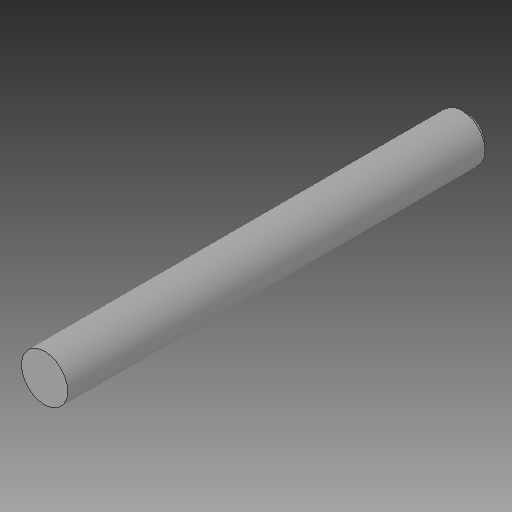
# Autodesk Inventor part: trappestift
Saved by Autodesk Inventor 2018 (Build 220112000, 112)
## iProperties
Created: 2019-09-29
Part Number: trappestift
Material: S355J2
Document SubType Name: Modeling
Designer: loppen
Density: 7.85 g/cm^3
Appearance: Light Gray
Mass: 876.014 g
Surface Area: 187.391 cm^2
Volume: 111.594 cm^3
Author: loppen
Autodesk Inventor part; units mm, degrees
ref_plane "YZ Plane" through (0, 0, 0) normal (1, 0, 0) x (0, 1, 0)
ref_plane "XZ Plane" through (0, 0, 0) normal (0, 1, 0) x (-1, 0, 0)
ref_plane "XY Plane" through (0, 0, 0) normal (0, 0, 1) x (1, 0, 0)
sketch "Sketch1" plane through (0, 0, 0) normal (0, 0, 1) x (1, 0, 0)
  circle A0 centre (0, 0) radius 12.5
  dimension "d0" = 25
  constraints: 1 centre point, 1 coincident
  measures "d0" diameter of A0
extrude "Extrusion1" add sketch "Sketch1" along normal blind 228
chamfer "Chamfer1" distance 3 angle 45 1 edges at (-12.5, 0, 0)
equation "\"d0\" = trappestifter_dia"
equation "\"d1\" = trappestifter_laengde"
equation "\"trappestifter_dia\" = 25"
equation "\"trappestifter_laengde\" = 228"
equation "\"perforeringsbredde\" = 6"
equation "\"perforeringshullaengde\" = 62.8"
equation "\"perforeringsoffset\" = 8"
equation "\"perforeringsoffset_top\" = 8"
equation "\"perforeringsoffset_bund\" = 8"
equation "\"laskehul_dia\" = 13"
equation "\"perforeringshullaengde_bund\" = 61.6"
equation "\"perforeringshullaengde_top\" = 61"
equation "\"trappestifter_huldia\" = 25.8"
equation "\"trappestifter_skraa_huldia\" = 26.6"
equation "\"trappevinkel\" = 34.3deg"
equation "\"balusterhul_udvidelse\" = 1"
equation "\"pladetykkelse\" = 3"
body "Solid1"
